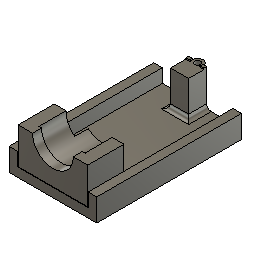
boring head jig v3 (Autodesk Fusion 360 design; units mm, degrees)
Autodesk Fusion 360 part; units mm, degrees
sketch "Sketch1" plane through (0, 0, 0) normal (0, 0, 1) x (1, 0, 0)
  circle A0 centre (0, 0) radius 25.5
  line L0 (-38.5, 0) -> (38.5, 0)
  line L1 (38.5, 0) -> (38.5, -40)
  line L2 (38.5, -40) -> (-38.5, -40)
  line L3 (-38.5, -40) -> (-38.5, 0)
  circle A1 centre (0, 0) radius 22.5
  dimension "d1" = 51
  dimension "d2" = 77
  dimension "d3" = 38.5
  dimension "d4" = 40
  dimension "d5" = 40
  dimension "d8" = 45
  constraint coincident A0.centre A1.centre
  constraint horizontal L0
  constraint vertical L1
  constraint horizontal L2
  constraint vertical L3
  constraint concentric A0 A1
  measures "d1" diameter of A0
  measures "d2" distance of L0.start L0.end
  measures "d3" distance of A0.centre L0.start
  measures "d4" distance of L0.end L1.end
  measures "d5" distance of A0.centre L2
  measures "d8" diameter of A1
extrude "Extrude1" add sketch "Sketch1" against normal blind 30 contours A0 L0 L1 L2 L3 makes body 1
extrude "Extrude2" add sketch "Sketch1" along normal blind 10 contours A0 L0 L1 L2 L3 | A0 L0 A1 picked at (-24.3213, -2.3847) bodies 1
sketch "Sketch2" plane through (0, 0, 10) normal (0, 0, 1) x (1, 0, 0)
  line L0 (-38.5, 0) -> (-38.5, -40)
  line L1 (-38.5, -40) -> (38.5, -40)
  line L2 (38.5, -40) -> (38.5, 0)
  line L3 (38.5, 0) -> (22.5, 0)
  arc A0 (-22.5, 0) -> (22.5, 0) centre (0, 0) ccw
  line L4 (-22.5, 0) -> (-38.5, 0)
  line L5 (-38.5, 0) -> (-38.5, -40)
  line L6 (-38.5, -40) -> (38.5, -40)
  line L7 (38.5, -40) -> (38.5, 0)
  line L8 (-39, 0) -> (-39, -40.5)
  line L9 (-39, -40.5) -> (39, -40.5)
  line L10 (39, -40.5) -> (39, 0)
  line L11 (-39, -25.5) -> (-48.5, -25.5)
  line L12 (-48.5, -25.5) -> (-48.5, -50.5)
  line L13 (-48.5, -50.5) -> (48.5, -50.5)
  line L14 (39, -25.5) -> (48.5, -25.5)
  line L15 (48.5, -25.5) -> (48.5, -50.5)
  dimension "d11" = 0.5
  dimension "d12" = 10
  dimension "d13" = 10
  dimension "d14" = 10
  dimension "d15" = 25
  dimension "d16" = 25
  constraint coincident L8 L11.start
  constraint perpendicular L8 L11
  constraint perpendicular L11 L12
  constraint perpendicular L12 L13
  constraint coincident L10 L14.start
  constraint perpendicular L10 L14
  constraint perpendicular L13 L15
  measures "d12" distance of L0.end L12
  measures "d13" distance of L1.end L15
  measures "d14" distance of L9 L13
  measures "d15" distance of L11.end L12.end
  measures "d16" distance of L13 L14
extrude "Extrude3" add sketch "Sketch2" against normal blind 160 separate body contours L8 L9 L10 L11 L12 L13 L14 L15 makes body 2
sketch "Sketch3" plane through (0, 0, -150) normal (0, 0, -1) x (-1, 0, 0)
  line L0 (48.5, -25.5) -> (39, -25.5)
  line L1 (39, -25.5) -> (39, -40.5)
  line L2 (39, -40.5) -> (-39, -40.5)
  line L3 (-39, -40.5) -> (-39, -25.5)
  line L4 (-39, -25.5) -> (-48.5, -25.5)
  line L5 (-48.5, -25.5) -> (-48.5, -50.5)
  line L6 (-48.5, -50.5) -> (48.5, -50.5)
  line L7 (48.5, -50.5) -> (48.5, -25.5)
  line L8 (-48.5, -50.5) -> (47.5, -50.5)
  line L9 (47.5, -50.5) -> (47.5, 0.1635)
  line L10 (47.5, 0.1635) -> (-48.5, 0.1635)
  line L11 (-48.5, 0.1635) -> (-48.5, -50.5)
  line L12 (-48.5, -1.3365) -> (47.5, -1.3365)
  line L13 (0, -50.5) -> (0, 0)
  line L14 (10, -50.5) -> (10, 0)
  line L15 (-10, -50.5) -> (-10, 0)
  line L16 (-10, 0) -> (10, 0)
  line L17 (10, 0) -> (10, -1.3365)
  line L18 (10, -1.3365) -> (-10, -1.3365)
  line L19 (-10, -1.3365) -> (-10, 0)
  dimension "d19" = 1.5
  dimension "d20" = 10
  dimension "d21" = -10
  constraint horizontal L8
  constraint vertical L9
  constraint horizontal L10
  constraint vertical L11
  constraint coincident L5.end L6.start
  constraint coincident L11 L12.start
  constraint coincident L9 L12.end
  constraint perpendicular L9 L12
  constraint midpoint L6 L13.start
  constraint coincident L13.end origin
  constraint horizontal L16
  constraint vertical L17
  constraint horizontal L18
  constraint vertical L19
  constraint coincident L14 L17.end
  constraint coincident L12 L17.end
  measures "d19" distance of L10 L12
extrude "Extrude4" add sketch "Sketch3" against normal blind 20 contours L2 L12 L13 L14 L18 | L2 L12 L13 L15 L18 bodies 2
extrude "Extrude5" add sketch "Sketch3" against normal blind 3 contours L12 L13 L14 L16 L17 L18 | L12 L13 L15 L16 L18 L19 bodies 2
sketch "Sketch4" plane through (0, -1.3365, 0) normal (0, 1, 0) x (-1, 0, 0)
  line L0 (-10, -147) -> (10, -147)
  line L1 (10, -147) -> (10, -130)
  line L2 (10, -130) -> (-10, -130)
  line L3 (-10, -130) -> (-10, -147)
  circle A0 centre (0, -150) radius 6
  circle A1 centre (0, -150) radius 3.2
  circle A2 centre (0, -150) radius 3.5
  dimension "d26" = 12
  dimension "d27" = 6.4
  dimension "d28" = 7
  constraint concentric A0 A1
  constraint concentric A1 A2
  measures "d26" diameter of A0
  measures "d27" diameter of A1
  measures "d28" diameter of A2
extrude "Extrude6" add sketch "Sketch4" against normal up to surface (49.1635 mm away) contours L0 A0 A2 | L0 A1 A2 picked at (-4.6502, -147.7734) picked at (-3.2989, -150.7958) bodies 2
extrude "Extrude7" cut sketch "Sketch4" against normal up to surface (49.1635 mm away) contours L0 A1 | L0 A1 bodies 2
extrude "Extrude8" cut sketch "Sketch4" along normal blind 6 contours L0 A0 A2 | L0 A0 A2 | L0 A1 A2 | L0 A1 A2 | L0 A1 | L0 A1 bodies 2
fillet "Fillet1" radius 5 3 edges at (0, -40.5, -130) (-10, -40.5, -140) (10, -40.5, -140) on bodies 2
sketch "Sketch5" plane through (0, 0, -30) normal (0, 0, -1) x (-1, 0, 0)
  line L0 (-38.5, -40) -> (38.5, -40)
  line L1 (38.5, -40) -> (38.5, 0)
  line L2 (38.5, 0) -> (25.5, 0)
  arc A0 (-25.5, 0) -> (25.5, 0) centre (0, 0) ccw
  line L3 (-25.5, 0) -> (-38.5, 0)
  line L4 (-38.5, 0) -> (-38.5, -40)
  arc A1 (-25.5, 0) -> (25.5, 0) centre (0, 0) ccw
  line L5 (-38.5, -40) -> (38.5, -40)
  line L6 (0, -40) -> (0, -25.5) construction
  line L7 (-16, -19.8557) -> (-16, -40)
  line L8 (16, -19.8557) -> (16, -40)
  dimension "d38" = 16
  constraint midpoint L5 L6.start
  constraint midpoint A0 L6.end
  constraint coincident A0 L7.start
  constraint coincident L0 L7.end
  constraint perpendicular L0 L7
  constraint symmetric L6 L7.start L8.start
  constraint symmetric L6 L7.end L8.end
  measures "d38" distance of L6.start L7.end
extrude "Extrude9" add sketch "Sketch5" along normal blind 15 contours L0 A0 A1 L5 L7 L8 bodies 1
equation "d3 = d2 / 2"
